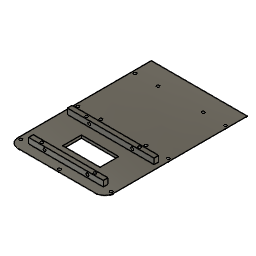
baseplate2 (Autodesk Fusion 360 design; units mm, degrees)
Autodesk Fusion 360 part; units mm, degrees
note: some values were not read from the file. Set by a fixed rule: which sketch regions a step uses.
sketch "Sketch1" plane through (0, 0, 0) normal (0, 0, 1) x (1, 0, 0)
  line L0 (0, 0) -> (-51.5, 0)
  line L1 (0, 0) -> (51.5, 0)
  line L2 (-51.5, 0) -> (-51.5, 265)
  line L3 (-51.5, 265) -> (51.5, 265)
  line L4 (51.5, 265) -> (51.5, 0)
  dimension "d1" = 51.5
  dimension "d2" = 51.5
  dimension "d3" = 265
  constraint coincident L0.start L1.start
  constraint horizontal L0
  constraint parallel L0 L1
  constraint perpendicular L0 L2
  constraint perpendicular L2 L3
  constraint perpendicular L1 L4
  measures "d1" distance of L0.start L0.end
  measures "d2" distance of L0.start L1.end
  measures "d3" distance of L0.end L2.end
extrude "Extrude1" add sketch "Sketch1" along normal blind 3
sketch "Sketch2" plane through (0, 0, 3) normal (0, 0, 1) x (-1, 0, 0)
  line L0 (51.5, 0) -> (-51.5, 0)
  line L1 (-51.5, 0) -> (-51.5, -265)
  line L2 (-51.5, -265) -> (51.5, -265)
  line L3 (51.5, -265) -> (51.5, 0)
  line L4 (0, 0) -> (0, -10)
  line L5 (0, -10) -> (46.5, -10)
  line L6 (0, -10) -> (-46.5, -10)
  line L7 (46.5, -10) -> (46.5, -15)
  line L8 (-46.5, -10) -> (-46.5, -15)
  line L9 (-46.5, -15) -> (46.5, -15)
  line L10 (0, -15) -> (0, -58)
  line L11 (0, -36.5) -> (25, -36.5)
  line L12 (-46.5, -58) -> (46.5, -58)
  line L13 (0, -63) -> (46.5, -63)
  line L14 (0, -63) -> (-46.5, -63)
  line L15 (46.5, -63) -> (46.5, -58)
  line L16 (-46.5, -63) -> (-46.5, -58)
  dimension "d6" = 10
  dimension "d7" = 46.5
  dimension "d8" = 46.5
  dimension "d9" = 5
  dimension "d10" = 43
  constraint coincident L4.start origin
  constraint perpendicular L0 L4
  constraint perpendicular L3 L5
  constraint perpendicular L4 L6
  constraint perpendicular L5 L7
  constraint perpendicular L6 L8
  constraint perpendicular L7 L9
  constraint midpoint L9 L10.start
  constraint perpendicular L9 L10
  constraint midpoint L10 L11.start
  constraint perpendicular L10 L11
  constraint symmetric L4.end L11 L13.start
  constraint symmetric L5.end L11 L13.end
  constraint symmetric L6.end L11 L14.end
  constraint symmetric L7.end L11 L12.end
  constraint symmetric L8.end L11 L12.start
  measures "d6" distance of L4.start L4.end
  measures "d7" distance of L4.end L5.end
  measures "d8" distance of L4.end L6.end
  measures "d9" distance of L5.end L7.end
  measures "d10" distance of L10.start L10.end
extrude "Extrude2" add sketch "Sketch2" along normal blind 6 contours L5 L6 L7 L8 L9 | L12 L13 L14 L15 L16
sketch "Sketch3" plane through (0, 10, 0) normal (0, -1, 0) x (1, 0, 0)
  line L0 (-46.5, 3) -> (46.5, 3)
  line L1 (46.5, 3) -> (46.5, 9)
  line L2 (46.5, 9) -> (-46.5, 9)
  line L3 (-46.5, 9) -> (-46.5, 3)
  line L4 (0, 9) -> (0, 6)
  line L5 (0, 6) -> (-23, 6)
  line L6 (0, 6) -> (23, 6)
  circle A0 centre (-23, 6) radius 1.5
  circle A1 centre (23, 6) radius 1.5
  dimension "d13" = 23
  dimension "d14" = 23
  dimension "d15" = 3
  dimension "d16" = 3
  constraint midpoint L2 L4.start
  constraint perpendicular L2 L4
  constraint perpendicular L4 L5
  constraint perpendicular L4 L6
  constraint coincident L5.end A0.centre
  constraint coincident L6.end A1.centre
  measures "d13" distance of L4.end L5.end
  measures "d14" distance of L4.end L6.end
  measures "d15" diameter of A0
  measures "d16" diameter of A1
extrude "Extrude3" cut sketch "Sketch3" against normal blind 53 contours A0 | A1
sketch "Sketch4" plane through (0, 0, 3) normal (0, 0, 1) x (-1, 0, 0)
  line L0 (46.5, -10) -> (46.5, -15)
  line L1 (46.5, -15) -> (-46.5, -15)
  line L2 (-46.5, -15) -> (-46.5, -10)
  line L3 (-46.5, -10) -> (46.5, -10)
  line L4 (-46.5, -63) -> (-46.5, -58)
  line L5 (-46.5, -58) -> (46.5, -58)
  line L6 (46.5, -58) -> (46.5, -63)
  line L7 (46.5, -63) -> (-46.5, -63)
  line L8 (51.5, 0) -> (-51.5, 0)
  line L9 (-51.5, 0) -> (-51.5, -265)
  line L10 (-51.5, -265) -> (51.5, -265)
  line L11 (51.5, -265) -> (51.5, 0)
  line L12 (0, -63) -> (0, -71.5)
  line L13 (-24.25, -71.5) -> (-24.25, -133)
  line L14 (-24.25, -133) -> (24.25, -133)
  line L15 (24.25, -133) -> (24.25, -74.5)
  circle A0 centre (24.25, -71.5) radius 1.5
  circle A1 centre (-24.25, -71.5) radius 1.5
  line L16 (-24.25, -71.5) -> (24.25, -71.5)
  circle A2 centre (-24.25, -133) radius 1.5
  circle A3 centre (24.25, -133) radius 1.5
  point P0 (24.25, -133)
  point P1 (-24.25, -133)
  dimension "d19" = 8.5
  dimension "d20" = 61.5
  dimension "d21" = 48.5
  dimension "d22" = 3
  dimension "d23" = 3
  dimension "d24" = 3
  dimension "d25" = 3
  constraint midpoint L7 L12.start
  constraint perpendicular L7 L12
  constraint perpendicular L13 L14
  constraint perpendicular L14 L15
  constraint coincident L13.start A1.centre
  constraint coincident P1 L13.end
  constraint coincident P0 L14.end
  constraint coincident A0.centre L16.end
  constraint perpendicular L13 L16
  measures "d19" distance of L12.start L12.end
  measures "d20" distance of L13.start P1
  measures "d21" distance of P1 P0
  measures "d22" diameter of A1
  measures "d23" diameter of A0
  measures "d24" diameter of A2
  measures "d25" diameter of A3
extrude "Extrude4" cut sketch "Sketch4" against normal blind 3 contours L13 A1 L16 | L13 A1 L16 | L13 L14 A2 | L13 L14 A2 | L14 L15 A3 | L14 L15 A3 | A0
sketch "Sketch5" plane through (0, 0, 3) normal (0, 0, 1) x (-1, 0, 0)
  circle A0 centre (-24.25, -133) radius 1.5
  circle A1 centre (24.25, -71.5) radius 1.5
  circle A2 centre (24.25, -133) radius 1.5
  circle A3 centre (-24.25, -71.5) radius 1.5
  line L0 (46.5, -10) -> (46.5, -15)
  line L1 (46.5, -15) -> (-46.5, -15)
  line L2 (-46.5, -15) -> (-46.5, -10)
  line L3 (-46.5, -10) -> (46.5, -10)
  line L4 (-46.5, -63) -> (-46.5, -58)
  line L5 (-46.5, -58) -> (46.5, -58)
  line L6 (46.5, -58) -> (46.5, -63)
  line L7 (46.5, -63) -> (-46.5, -63)
  line L8 (51.5, 0) -> (-51.5, 0)
  line L9 (-51.5, 0) -> (-51.5, -265)
  line L10 (-51.5, -265) -> (51.5, -265)
  line L11 (51.5, -265) -> (51.5, 0)
  line L12 (24.25, -133) -> (-24.25, -133)
  line L13 (0, -133) -> (0, -173)
  line L14 (0, -238) -> (-35, -238)
  line L15 (0, -238) -> (35, -238)
  line L16 (0, -233) -> (35, -233)
  line L17 (0, -233) -> (-35, -233)
  line L18 (0, -178) -> (35, -178)
  line L19 (0, -178) -> (-35, -178)
  line L20 (0, -173) -> (-35, -173)
  line L21 (0, -173) -> (35, -173)
  line L22 (-35, -178) -> (-35, -173)
  line L23 (35, -173) -> (35, -178)
  line L24 (35, -238) -> (35, -233)
  line L25 (-35, -238) -> (-35, -233)
  line L26 (0, -173) -> (-12.9802, -153.9099)
  dimension "d28" = 40
  dimension "d29" = 5
  constraint coincident A2.centre L12.start
  constraint coincident A0.centre L12.end
  constraint midpoint L12 L13.start
  constraint perpendicular L12 L13
  constraint perpendicular L20 L22
  constraint perpendicular L3 L23
  constraint perpendicular L16 L24
  constraint perpendicular L17 L25
  measures "d28" distance of L13.start L13.end
  measures "d29" distance of L13.end L18.start
extrude "Extrude5" add sketch "Sketch5" along normal blind 10 contours L14 L15 L16 L17 L24 L25 | L18 L19 L20 L21 L22 L23
sketch "Sketch6" plane through (0, 238, 0) normal (0, 1, 0) x (-1, 0, 0)
  line L0 (-35, 3) -> (35, 3)
  line L1 (35, 3) -> (35, 13)
  line L2 (35, 13) -> (-35, 13)
  line L3 (-35, 13) -> (-35, 3)
  line L4 (0, 13) -> (0, 3)
  line L5 (0, 8) -> (-22.5, 8)
  line L6 (0, 8) -> (22.5, 8)
  circle A0 centre (-22.5, 8) radius 2
  circle A1 centre (22.5, 8) radius 2
  dimension "d32" = 22.5
  dimension "d33" = 22.5
  dimension "d34" = 4
  dimension "d35" = 4
  constraint midpoint L2 L4.start
  constraint midpoint L0 L4.end
  constraint midpoint L4 L5.start
  constraint perpendicular L4 L5
  constraint perpendicular L4 L6
  constraint coincident L5.end A0.centre
  constraint coincident L6.end A1.centre
  measures "d32" distance of L5.start L5.end
  measures "d33" distance of L5.start L6.end
  measures "d34" diameter of A0
  measures "d35" diameter of A1
extrude "Extrude6" cut sketch "Sketch6" against normal blind 80 contours A0 | A1
sketch "Sketch7" plane through (0, 0, 3) normal (0, 0, 1) x (-1, 0, 0)
  line L0 (35, -173) -> (35, -178)
  line L1 (35, -178) -> (-35, -178)
  line L2 (-35, -178) -> (-35, -173)
  line L3 (-35, -173) -> (35, -173)
  line L4 (-35, -238) -> (-35, -233)
  line L5 (-35, -233) -> (35, -233)
  line L6 (35, -233) -> (35, -238)
  line L7 (35, -238) -> (-35, -238)
  circle A0 centre (-24.25, -133) radius 1.5
  circle A1 centre (24.25, -71.5) radius 1.5
  circle A2 centre (24.25, -133) radius 1.5
  circle A3 centre (-24.25, -71.5) radius 1.5
  line L8 (46.5, -10) -> (46.5, -15)
  line L9 (46.5, -15) -> (-46.5, -15)
  line L10 (-46.5, -15) -> (-46.5, -10)
  line L11 (-46.5, -10) -> (46.5, -10)
  line L12 (-46.5, -63) -> (-46.5, -58)
  line L13 (-46.5, -58) -> (46.5, -58)
  line L14 (46.5, -58) -> (46.5, -63)
  line L15 (46.5, -63) -> (-46.5, -63)
  line L16 (51.5, 0) -> (-51.5, 0)
  line L17 (-51.5, 0) -> (-51.5, -265)
  line L18 (-51.5, -265) -> (51.5, -265)
  line L19 (51.5, -265) -> (51.5, 0)
  line L20 (0, -238) -> (0, -248)
  line L21 (0, -248) -> (3, -248)
  line L22 (0, -248) -> (-3, -248)
  line L23 (0, -265) -> (0, -260)
  line L24 (3, -248) -> (3, -258)
  line L25 (3, -258) -> (8, -258)
  line L26 (3, -248) -> (8, -248)
  line L27 (8, -258) -> (8, -248)
  line L28 (-3, -248) -> (-3, -258)
  line L29 (-3, -258) -> (-8, -258)
  line L30 (-8, -258) -> (-8, -248)
  line L31 (-3, -248) -> (-8, -248)
  dimension "d38" = 10
  dimension "d39" = 3
  dimension "d40" = 3
  dimension "d41" = 5
  dimension "d42" = 10
  dimension "d43" = 5
  dimension "d44" = 5
  dimension "d45" = 5
  dimension "d46" = 10
  constraint midpoint L7 L20.start
  constraint perpendicular L7 L20
  constraint perpendicular L20 L21
  constraint perpendicular L20 L22
  constraint midpoint L18 L23.start
  constraint perpendicular L18 L23
  constraint perpendicular L21 L24
  constraint perpendicular L24 L25
  constraint perpendicular L20 L26
  constraint perpendicular L22 L28
  constraint perpendicular L28 L29
  constraint perpendicular L29 L30
  constraint perpendicular L30 L31
  measures "d38" distance of L20.start L20.end
  measures "d39" distance of L20.end L21.end
  measures "d40" distance of L20.end L22.end
  measures "d41" distance of L23.start L23.end
  measures "d42" distance of L21.end L24.end
  measures "d43" distance of L24.end L25.end
  measures "d44" distance of L21.end L26.end
  measures "d45" distance of L28.end L29.end
  measures "d46" distance of L29.end L30.end
extrude "Extrude7" add sketch "Sketch7" along normal blind 6 contours L24 L25 L26 L27 | L28 L29 L30 L31
sketch "Sketch8" plane through (8, 0, 0) normal (1, 0, 0) x (0, 1, 0)
  line L0 (248, 3) -> (258, 3)
  line L1 (258, 3) -> (258, 9)
  line L2 (258, 9) -> (248, 9)
  line L3 (248, 9) -> (248, 3)
  line L4 (253, 3) -> (253, 9)
  circle A0 centre (253, 6) radius 1.5
  dimension "d49" = 3
  constraint midpoint L0 L4.start
  constraint midpoint L2 L4.end
  constraint midpoint L4 A0.centre
  measures "d49" diameter of A0
extrude "Extrude8" cut sketch "Sketch8" against normal blind 20 contours L4 A0 | L4 A0
fillet "Fillet1" radius 10 4 edges at (51.5, 0, 1.5) (-51.5, 0, 1.5) (51.5, 265, 1.5) (-51.5, 265, 1.5)
fillet "Fillet2" radius 5 8 edges at (51.5, 132.5, 0) (48.5711, 262.0711, 0) (0, 265, 0) (-48.5711, 262.0711, 0) (-51.5, 132.5, 0) (-48.5711, 2.9289, 0) (0, 0, 0) (48.5711, 2.9289, 0)
sketch "Sketch9" plane through (0, 0, 3) normal (0, 0, 1) x (-1, 0, 0)
  arc A0 (41.5, -265) -> (51.5, -255) centre (41.5, -255) ccw
  line L0 (51.5, -255) -> (51.5, -10)
  arc A1 (51.5, -10) -> (41.5, 0) centre (41.5, -10) ccw
  line L1 (41.5, 0) -> (-41.5, 0)
  arc A2 (-41.5, 0) -> (-51.5, -10) centre (-41.5, -10) ccw
  line L2 (-51.5, -10) -> (-51.5, -255)
  arc A3 (-51.5, -255) -> (-41.5, -265) centre (-41.5, -255) ccw
  line L3 (-41.5, -265) -> (41.5, -265)
  line L4 (-3, -258) -> (-8, -258)
  line L5 (-8, -258) -> (-8, -248)
  line L6 (-8, -248) -> (-3, -248)
  line L7 (-3, -248) -> (-3, -258)
  line L8 (3, -248) -> (8, -248)
  line L9 (8, -248) -> (8, -258)
  line L10 (8, -258) -> (3, -258)
  line L11 (3, -258) -> (3, -248)
  line L12 (35, -173) -> (35, -178)
  line L13 (35, -178) -> (-35, -178)
  line L14 (-35, -178) -> (-35, -173)
  line L15 (-35, -173) -> (35, -173)
  line L16 (-35, -238) -> (-35, -233)
  line L17 (-35, -233) -> (35, -233)
  line L18 (35, -233) -> (35, -238)
  line L19 (35, -238) -> (-35, -238)
  circle A4 centre (-24.25, -133) radius 1.5
  circle A5 centre (24.25, -71.5) radius 1.5
  circle A6 centre (24.25, -133) radius 1.5
  circle A7 centre (-24.25, -71.5) radius 1.5
  line L20 (46.5, -10) -> (46.5, -15)
  line L21 (46.5, -15) -> (-46.5, -15)
  line L22 (-46.5, -15) -> (-46.5, -10)
  line L23 (-46.5, -10) -> (46.5, -10)
  line L24 (-46.5, -63) -> (-46.5, -58)
  line L25 (-46.5, -58) -> (46.5, -58)
  line L26 (46.5, -58) -> (46.5, -63)
  line L27 (46.5, -63) -> (-46.5, -63)
  line L28 (0, -58) -> (0, -15)
  line L29 (0, -36.5) -> (20, -36.5)
  line L30 (0, -36.5) -> (-20, -36.5)
  line L31 (20, -36.5) -> (20, -46.5)
  line L32 (-20, -36.5) -> (-20, -46.5)
  line L33 (20, -46.5) -> (-20, -46.5)
  line L34 (20, -36.5) -> (20, -26.5)
  line L35 (20, -26.5) -> (-20, -26.5)
  line L36 (-20, -36.5) -> (-20, -26.5)
  dimension "d56" = 20
  dimension "d57" = 20
  dimension "d58" = 10
  dimension "d59" = 10
  dimension "d60" = 10
  dimension "d61" = 40
  constraint midpoint L25 L28.start
  constraint midpoint L21 L28.end
  constraint midpoint L28 L29.start
  constraint perpendicular L28 L29
  constraint perpendicular L28 L30
  constraint perpendicular L25 L31
  constraint perpendicular L30 L32
  constraint perpendicular L29 L34
  constraint perpendicular L28 L35
  measures "d56" distance of L29.start L29.end
  measures "d57" distance of L29.start L30.end
  measures "d58" distance of L29.end L31.end
  measures "d59" distance of L30.end L32.end
  measures "d60" distance of L29.end L34.end
  measures "d61" distance of L34.end L35.end
extrude "Extrude9" cut sketch "Sketch9" against normal blind 5 contours L28 L30 L32 L33 | L28 L29 L31 L33 | L28 L30 L35 L36 | L28 L29 L34 L35
sketch "Sketch10" plane through (0, 0, 9) normal (0, 0, 1) x (-1, 0, 0)
  line L0 (-46.5, -63) -> (46.5, -63)
  line L1 (46.5, -63) -> (46.5, -58)
  line L2 (46.5, -58) -> (-46.5, -58)
  line L3 (-46.5, -58) -> (-46.5, -63)
  line L4 (46.5, -60.5) -> (28.5, -60.5)
  circle A0 centre (28.5, -60.5) radius 1.5
  line L5 (0, -58) -> (0, -50)
  line L6 (46.5, -58) -> (46.5, -15)
  line L7 (46.5, -36.5) -> (70, -36.5)
  circle A1 centre (28.5, -12.5) radius 1.5
  circle A2 centre (-28.5, -60.5) radius 1.5
  circle A3 centre (-28.5, -12.5) radius 1.5
  point P0 (28.5, -12.5)
  dimension "d64" = 18
  dimension "d65" = 3
  dimension "d66" = 3
  constraint midpoint L1 L4.start
  constraint perpendicular L1 L4
  constraint coincident L4.end A0.centre
  constraint midpoint L2 L5.start
  constraint perpendicular L2 L5
  constraint coincident L1.end L2.start
  constraint perpendicular L2 L6
  constraint midpoint L6 L7.start
  constraint perpendicular L6 L7
  constraint symmetric L4.end L7 P0
  constraint coincident P0 A1.centre
  constraint symmetric A0 L5 A2
  constraint symmetric L5 A1 A3
  measures "d64" distance of L4.start L4.end
  measures "d65" diameter of A0
  measures "d66" diameter of A1
extrude "Extrude10" cut sketch "Sketch10" against normal blind 50 contours A0 | A1 | A2 | A3
sketch "Sketch11" plane through (0, 0, 3) normal (0, 0, 1) x (-1, 0, 0)
  line L0 (-20, -26.5) -> (20, -26.5)
  line L1 (20, -26.5) -> (20, -46.5)
  line L2 (20, -46.5) -> (-20, -46.5)
  line L3 (-20, -46.5) -> (-20, -26.5)
  arc A0 (41.5, -265) -> (51.5, -255) centre (41.5, -255) ccw
  line L4 (51.5, -255) -> (51.5, -10)
  arc A1 (51.5, -10) -> (41.5, 0) centre (41.5, -10) ccw
  line L5 (41.5, 0) -> (-41.5, 0)
  arc A2 (-41.5, 0) -> (-51.5, -10) centre (-41.5, -10) ccw
  line L6 (-51.5, -10) -> (-51.5, -255)
  arc A3 (-51.5, -255) -> (-41.5, -265) centre (-41.5, -255) ccw
  line L7 (-41.5, -265) -> (41.5, -265)
  line L8 (-3, -258) -> (-8, -258)
  line L9 (-8, -258) -> (-8, -248)
  line L10 (-8, -248) -> (-3, -248)
  line L11 (-3, -248) -> (-3, -258)
  line L12 (3, -248) -> (8, -248)
  line L13 (8, -248) -> (8, -258)
  line L14 (8, -258) -> (3, -258)
  line L15 (3, -258) -> (3, -248)
  line L16 (35, -173) -> (35, -178)
  line L17 (35, -178) -> (-35, -178)
  line L18 (-35, -178) -> (-35, -173)
  line L19 (-35, -173) -> (35, -173)
  line L20 (-35, -238) -> (-35, -233)
  line L21 (-35, -233) -> (35, -233)
  line L22 (35, -233) -> (35, -238)
  line L23 (35, -238) -> (-35, -238)
  circle A4 centre (-24.25, -133) radius 1.5
  circle A5 centre (24.25, -71.5) radius 1.5
  circle A6 centre (24.25, -133) radius 1.5
  circle A7 centre (-24.25, -71.5) radius 1.5
  line L24 (46.5, -10) -> (46.5, -15)
  line L25 (46.5, -15) -> (-46.5, -15)
  line L26 (-46.5, -15) -> (-46.5, -10)
  line L27 (-46.5, -10) -> (46.5, -10)
  line L28 (-46.5, -63) -> (-46.5, -58)
  line L29 (-46.5, -58) -> (46.5, -58)
  line L30 (46.5, -58) -> (46.5, -63)
  line L31 (46.5, -63) -> (-46.5, -63)
  line L32 (51.5, -255) -> (48.5, -255)
  circle A8 centre (48.5, -255) radius 1.5
  line L33 (51.5, -132.5) -> (48.5, -132.5)
  circle A9 centre (48.5, -132.5) radius 1.5
  line L34 (48.5, -255) -> (48.5, -132.5)
  circle A10 centre (48.5, -193.75) radius 1.5
  line L35 (0, -265) -> (0, -262)
  circle A11 centre (0, -262) radius 1.5
  circle A12 centre (0, -3) radius 1.5
  circle A13 centre (48.5, -10) radius 1.5
  circle A14 centre (48.5, -71.25) radius 1.5
  circle A15 centre (48.5, -132.5) radius 1.5
  circle A16 centre (-48.5, -10) radius 1.5
  circle A17 centre (-48.5, -71.25) radius 1.5
  circle A18 centre (-48.5, -132.5) radius 1.5
  circle A19 centre (-48.5, -193.75) radius 1.5
  circle A20 centre (-48.5, -255) radius 1.5
  dimension "d69" = 3
  dimension "d70" = 3
  dimension "d71" = 3
  dimension "d72" = 3
  dimension "d73" = 3
  dimension "d74" = 3
  dimension "d75" = 3
  constraint coincident A0.end L4.start
  constraint perpendicular L4 L32
  constraint coincident L32.end A8.centre
  constraint midpoint L4 L33.start
  constraint perpendicular L4 L33
  constraint coincident L33.end A9.centre
  constraint midpoint L34 A10.centre
  constraint midpoint L7 L35.start
  constraint perpendicular L7 L35
  constraint coincident L35.end A11.centre
  constraint symmetric A8 L33 A13
  constraint symmetric L33 A9 A15
  constraint symmetric L33 A10 A14
  constraint symmetric L33 A11 A12
  constraint symmetric A8 L35 A20
  constraint symmetric A10 L35 A19
  constraint symmetric L35 A13 A16
  constraint symmetric L35 A14 A17
  constraint symmetric L35 A15 A18
  measures "d69" distance of A0.end L32.end
  measures "d70" diameter of A8
  measures "d71" distance of L33.start L33.end
  measures "d72" diameter of A9
  measures "d73" diameter of A10
  measures "d74" distance of L35.start L35.end
  measures "d75" diameter of A11
extrude "Extrude11" cut sketch "Sketch11" against normal blind 5 contours L32 A8 L34 | L32 A8 L34 | L33 A9 L34 A15 | L33 A9 L34 A15 | L34 A10 | L34 A10 | A11 | A12 | A13 | A14 | A16 | A17 | A18 | A19 | A20
sketch "Sketch12" plane through (0, 0, 3) normal (0, 0, 1) x (-1, 0, 0)
  circle A0 centre (48.5, -255) radius 1.5
  circle A1 centre (-48.5, -193.75) radius 1.5
  circle A2 centre (-48.5, -10) radius 1.5
  circle A3 centre (48.5, -10) radius 1.5
  circle A4 centre (-48.5, -132.5) radius 1.5
  circle A5 centre (0, -262) radius 1.5
  circle A6 centre (48.5, -193.75) radius 1.5
  circle A7 centre (-48.5, -71.25) radius 1.5
  circle A8 centre (0, -3) radius 1.5
  circle A9 centre (48.5, -71.25) radius 1.5
  circle A10 centre (48.5, -132.5) radius 1.5
  circle A11 centre (-48.5, -255) radius 1.5
  line L0 (-20, -26.5) -> (20, -26.5)
  line L1 (20, -26.5) -> (20, -46.5)
  line L2 (20, -46.5) -> (-20, -46.5)
  line L3 (-20, -46.5) -> (-20, -26.5)
  arc A12 (41.5, -265) -> (51.5, -255) centre (41.5, -255) ccw
  line L4 (51.5, -255) -> (51.5, -10)
  arc A13 (51.5, -10) -> (41.5, 0) centre (41.5, -10) ccw
  line L5 (41.5, 0) -> (-41.5, 0)
  arc A14 (-41.5, 0) -> (-51.5, -10) centre (-41.5, -10) ccw
  line L6 (-51.5, -10) -> (-51.5, -255)
  arc A15 (-51.5, -255) -> (-41.5, -265) centre (-41.5, -255) ccw
  line L7 (-41.5, -265) -> (41.5, -265)
  line L8 (-3, -258) -> (-8, -258)
  line L9 (-8, -258) -> (-8, -248)
  line L10 (-8, -248) -> (-3, -248)
  line L11 (-3, -248) -> (-3, -258)
  line L12 (3, -248) -> (8, -248)
  line L13 (8, -248) -> (8, -258)
  line L14 (8, -258) -> (3, -258)
  line L15 (3, -258) -> (3, -248)
  line L16 (35, -173) -> (35, -178)
  line L17 (35, -178) -> (-35, -178)
  line L18 (-35, -178) -> (-35, -173)
  line L19 (-35, -173) -> (35, -173)
  line L20 (-35, -238) -> (-35, -233)
  line L21 (-35, -233) -> (35, -233)
  line L22 (35, -233) -> (35, -238)
  line L23 (35, -238) -> (-35, -238)
  circle A16 centre (-24.25, -133) radius 1.5
  circle A17 centre (24.25, -71.5) radius 1.5
  circle A18 centre (24.25, -133) radius 1.5
  circle A19 centre (-24.25, -71.5) radius 1.5
  line L24 (46.5, -10) -> (46.5, -15)
  line L25 (46.5, -15) -> (-46.5, -15)
  line L26 (-46.5, -15) -> (-46.5, -10)
  line L27 (-46.5, -10) -> (46.5, -10)
  line L28 (-46.5, -63) -> (-46.5, -58)
  line L29 (-46.5, -58) -> (46.5, -58)
  line L30 (46.5, -58) -> (46.5, -63)
  line L31 (46.5, -63) -> (-46.5, -63)
  line L32 (0, -173) -> (0, -133)
  line L33 (0, -153) -> (51.5, -153)
  line L34 (0, -153) -> (-51.5, -153)
  line L35 (-51.5, -153) -> (-51.5, -280)
  line L36 (-51.5, -280) -> (51.5, -280)
  line L37 (51.5, -280) -> (51.5, -153)
  line L38 (-51.5, -153) -> (-51.5, 0)
  line L39 (-51.5, 0) -> (51.5, 0)
  line L40 (51.5, 0) -> (51.5, -153)
  constraint midpoint L19 L32.start
  constraint perpendicular L19 L32
  constraint midpoint L32 L33.start
  constraint coincident L4 L33.end
  constraint perpendicular L4 L33
  constraint coincident L6 L34.end
  constraint perpendicular L6 L34
  constraint perpendicular L34 L35
  constraint perpendicular L4 L36
  constraint perpendicular L33 L37
  constraint perpendicular L34 L38
  constraint perpendicular L4 L39
  constraint perpendicular L33 L40
sketch "Sketch16" plane through (0, 0, 9) normal (0, 0, 1) x (-1, 0, 0)
  circle A0 centre (-28.5, -12.5) radius 1.5
  circle A1 centre (28.5, -12.5) radius 1.5
  line L0 (46.5, -10) -> (-46.5, -10)
  line L1 (-46.5, -10) -> (-46.5, -15)
  line L2 (-46.5, -15) -> (46.5, -15)
  line L3 (46.5, -15) -> (46.5, -10)
  line L4 (46.5, -15) -> (40, -15)
  line L5 (40, -15) -> (40, -10)
  line L6 (40, -10) -> (46.5, -10)
  line L7 (46.5, -10) -> (46.5, -15)
  line L8 (-46.5, -15) -> (-40, -15)
  line L9 (-46.5, -10) -> (-40, -10)
  line L10 (-40, -10) -> (-40, -15)
  dimension "d82" = 6.5
  dimension "d83" = 6.5
  constraint coincident L2.end L3.start
  constraint perpendicular L3 L4
  constraint perpendicular L4 L5
  constraint coincident L0.start L3.end
  constraint perpendicular L3 L6
  constraint coincident L1.end L2.start
  constraint perpendicular L1 L8
  constraint coincident L0.end L1.start
  constraint coincident L0 L9.end
  constraint perpendicular L1 L9
  measures "d82" distance of L2.end L4.end
  measures "d83" distance of L1.end L8.end
extrude "Extrude13" cut sketch "Sketch16" against normal blind 6 contours L0 L2 L3 L4 L5 L6 L7 | L0 L1 L2 L8 L9 L10
extrude "Extrude12" cut sketch "Sketch12" along normal blind 10 and the other way blind 40 contours A12 L4 L6 A15 L7 L33 L34 L35 L37 | L8 L9 L10 L11 | L12 L13 L14 L15 | L16 L17 L18 L19 | L20 L21 L22 L23
